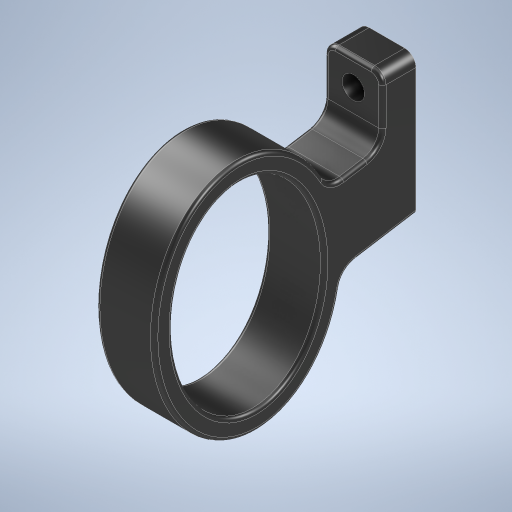
# Autodesk Inventor part: TorsoBackBumper
Saved by Autodesk Inventor 2024.2 (Build 282272000, 272)
## iProperties
Created: 2024-01-21
Part Number: TorsoBackBumper
Material: ABS Plastic
Document SubType Name: Modeling
Designer: Masato Kubotera
Density: 1.06 g/cm^3
Appearance: Glossy - Black
Mass: 18.7145 g
Surface Area: 72.9359 cm^2
Volume: 17.6552 cm^3
Catalog Web Link: https://www.poly-maker.jp/polyflex-tpu90.html
Author: Masato Kubotera
Autodesk Inventor part; units mm, degrees
ref_plane "YZ Plane" through (0, 0, 0) normal (1, 0, 0) x (0, 1, 0)
ref_plane "XZ Plane" through (0, 0, 0) normal (0, 1, 0) x (-1, 0, 0)
ref_plane "XY Plane" through (0, 0, 0) normal (0, 0, 1) x (1, 0, 0)
sketch "Sketch1" plane through (0, 0, 0) normal (0, 1, 0) x (-1, 0, 0)
  line L0 (0, -16) -> (0, 16)
  line L1 (0, 16) -> (-9, 16)
  line L2 (0, 9) -> (-9, 9) construction
  line L3 (0, 0) -> (-42.387, 0) construction
  line L4 (0, -9) -> (-21.1341, -9) construction
  line L5 (0, -16) -> (0, -21)
  line L6 (0, -21) -> (-19.7389, -24.2072)
  line L7 (-23.0963, -3.5435) -> (-13.1981, -1.9353)
  line L8 (0, 16) -> (5, 16) construction
  line L9 (5, 16) -> (5, -16) construction
  line L10 (5, -16) -> (0, -16) construction
  line L11 (-25.038, -14.4636) -> (63.9802, 0) construction
  ellipse E0 centre (-44.7791, -17.6711) end of major axis (-39.5669, -49.7504) minor radius 25
  line L12 (-49.9913, 14.4082) -> (-49.1895, 9.4729) construction
  line L13 (-9, 16) -> (-9, 3)
  arc A0 (-13.1981, -1.9353) -> (-9, 3) centre (-14, 3) ccw
  line L14 (-13.1981, -1.9353) -> (-9, -1.2532)
  line L15 (-9, 3) -> (-9, -1.2532)
  line L16 (-70, 16) -> (-70, -14.9643) construction
  ellipse E1 centre (-44.7791, -17.6711) end of major axis (-49.1895, 9.4729) minor radius 20
  line L17 (-42.6675, -50) -> (-70, -50) construction
  line L18 (-49.9913, 14.4082) -> (-39.5669, -49.7504) construction
  point P0 (-19.1571, -6.9591)
  point P1 (-5.8036, -25.2394)
  dimension "d34" = 25
  dimension "d45" = 20
  dimension "d1" = 9
  dimension "d2" = 18
  dimension "d21" = 5
  dimension "d22" = 5
  dimension "d23" = 32
  dimension "d40" = 5
  dimension "d42" = 70
  dimension "d44" = 5
  dimension "d46" = 6
  dimension "d47" = 50
  dimension "d51" = 65
  constraints: 38 end point, 9 point on line, 7 horizontal, 5 vertical, 3 perpendicular, 2 point on circle, 2 symmetric about line, 2 tangent, 1 centre point, 1 coincident, 1 collinear, 1 midpoint, 1 parallel, 17 other
  measures "d1" distance of L2.end L2.start
  measures "d2" distance of L4.start L2.start
  measures "d21" distance of L0.end L8.end
  measures "d22" distance of L0.start L5.end
  measures "d23" distance of L8.end L9.end
  measures "d40" radius of A0
  measures "d42" distance between parallel lines of L0 L16
  measures "d44" distance of L12.start L12.end
  measures "d46" distance from line of L13.end L2
  measures "d47" distance between parallel lines of L17 L3
  measures "d51" distance of L12.start L18.end
extrude "Extrusion1" add sketch "Sketch1" along normal blind 15.5
sketch "Sketch3" plane through (0, 0, -21) normal (-1, 0, 0) x (0, 0, 1)
  line L0 (0, 15.5) -> (37, 15.5) projected
  line L1 (30, 15.5) -> (30, 0)
  line L2 (12, 15.5) -> (12, 0)
  point P0 (21, 0)
  point P1 (12, 0)
  point P2 (30, 7.75)
  point P3 (12, 7.75)
  constraints: 4 end point, 2 coincident, 2 midpoint, 2 point on line, 2 vertical
hole "Hole2" at (0, 7.75, 9) at (0, 7.75, -9) direction (1, 0, 0) diameter 6 depth 9
fillet "Fillet1" radius 5 2 edges at (19.7389, 7.75, -24.2072) (23.0963, 7.75, -3.5435)
fillet "Fillet2" radius 1 17 edges at (16.3308, 15.5, -2.4443) (10.1915, 15.5, -0.2396) (9, 15.5, 9.5) (9, 7.75, 16) (9, 0, 9.5) (10.1915, 0, -0.2396) (16.3308, 0, -2.4443) (22.4474, 0, -2.5168) (69.4555, 0, -21.6805) (18.7983, 0, -24.9756) (8.0531, 0, -22.3085) (69.4555, 15.5, -21.6805) (18.7983, 15.5, -24.9756) (8.0531, 15.5, -22.3085) (22.4474, 15.5, -2.5168) (40.3688, 15.5, -44.8151) (40.3688, 0, -44.8151)
chamfer "Chamfer1" distance 1 angle 45 2 edges at (0, 7.75, -12) (0, 7.75, 6)
fillet "Fillet3" radius 3 4 edges at (8.7071, 15.2071, 15.7071) (4, 15.5, 16) (8.7071, 0.2929, 15.7071) (4, 0, 16)
body "Solid1"
